joint (Autodesk Fusion 360 design; units mm, degrees)
Autodesk Fusion 360 part; units mm, degrees
sketch "Sketch1" plane through (0, 0, 0) normal (0, 0, 1) x (1, 0, 0)
  line L0 (7.5, -6.5) -> (-7.5, -6.5)
  line L1 (-7.5, -6.5) -> (-7.5, 7.5)
  line L2 (-7.5, 7.5) -> (7.5, 7.5)
  line L3 (7.5, 7.5) -> (7.5, -6.5)
  circle A0 centre (0, 0) radius 3.75
  dimension "d1" = 15
  dimension "d3" = 7.5
  dimension "d4" = 7.5
  dimension "d5" = 6.5
  constraint horizontal L0
  constraint perpendicular L0 L1
  constraint parallel L0 L2
  constraint parallel L1 L3
  constraint coincident A0.centre origin
  measures "d1" distance of L1.end L2.end
  measures "d3" diameter of A0
  measures "d4" distance of L2 A0.centre
  measures "d5" distance of L0 A0.centre
extrude "Extrude1" add sketch "Sketch1" along normal blind 15 makes body 1
fillet "Fillet1" radius 7.5 2 edges at (-7.5, -6.5, 7.5) (7.5, -6.5, 7.5) on bodies 1
mirror "Mirror1" about plane through (-7.5, 7.5, 0) normal (0, 1, 0) of bodies 1 makes body 2
move_body "Move1" bodies 2 to x (0, 0, 1) y (0, 1, 0) z (-1, 0, 0) at (0, 0, 0)
move_body "Move2" bodies 2 to x (1, 0, 0) y (0, 1, 0) z (0, 0, 1) at (7.5, 0, 7.5)
combine "Combine1" operation add target body 2 tool bodies 1
fillet "Fillet2" radius 2 8 edges at (7.5, 21.5, 7.5) (7.5, 7.5, 0) (0, -6.5, 0) (-7.5, 7.5, 0) (-7.5, 21.5, 7.5) (-7.5, 7.5, 15) (0, -6.5, 15) (7.5, 7.5, 15) on bodies 2
equation "d3 = ( 15 / 2 ) * 1 mm"
